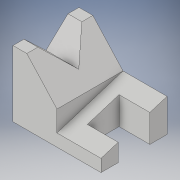
# Autodesk Inventor part: orthographic2
Saved by Autodesk Inventor 2017 (Build 210142000, 142)
## iProperties
Created: 2018-11-30
Part Number: orthographic2
Material: Generic
Document SubType Name: Modeling
Designer: qthuynh
Density: 1 g/cm^3
Appearance: Default
Author: qthuynh
Autodesk Inventor part; units mm, degrees
ref_plane "YZ Plane" through (0, 0, 0) normal (1, 0, 0) x (0, 1, 0)
ref_plane "XZ Plane" through (0, 0, 0) normal (0, 1, 0) x (-1, 0, 0)
ref_plane "XY Plane" through (0, 0, 0) normal (0, 0, 1) x (1, 0, 0)
sketch "Sketch1" plane through (0, 0, 0) normal (0, 0, 1) x (1, 0, 0)
  line L0 (0, 0) -> (101.6, 0)
  line L1 (101.6, 0) -> (101.6, 76.2)
  line L2 (101.6, 76.2) -> (0, 76.2)
  line L3 (0, 76.2) -> (0, 0)
  dimension "d0" = 101.6
  dimension "d1" = 76.2
  constraints: 8 end point, 2 parallel, 1 horizontal, 1 perpendicular
  measures "d0" distance of L2.end L1.end
  measures "d1" distance of L1.end L0.end
extrude "Extrusion1" add sketch "Sketch1" along normal blind 76.2
sketch "Sketch2" plane through (0, 76.2, 0) normal (0, 1, 0) x (1, 0, 0)
  line L0 (101.6, 0) -> (101.6, -76.2) projected
  line L1 (101.6, -19.812) -> (66.04, -19.812)
  line L2 (66.04, -19.812) -> (66.04, -56.388)
  line L3 (66.04, -56.388) -> (101.6, -56.388)
  line L4 (101.6, -56.388) -> (101.6, -19.812)
  point P0 (0, 0)
  dimension "d4" = 35.56
  dimension "d5" = 36.576
  dimension "d6" = 19.812
  constraints: 8 end point, 2 parallel, 1 horizontal, 1 perpendicular, 1 point on line
  measures "d4" distance of L3.end L2.end
  measures "d5" distance of L2.end L1.end
  measures "d6" distance of L0.start L1.start
extrude "Extrusion2" cut sketch "Sketch2" against normal blind 76.2
sketch "Sketch3" plane through (0, 0, 76.2) normal (0, 0, 1) x (1, 0, 0)
  line L0 (0, 75.8832) -> (15.9989, 76.2)
  line L1 (101.6, 76.2) -> (0, 76.2) projected
  line L2 (66.04, 0) -> (101.6, 0) projected
  line L3 (101.6, 0) -> (50.8, 0)
  line L4 (101.6, 0) -> (101.6, 38.1)
  line L5 (101.6, 76.2) -> (101.6, 0) projected
  line L6 (50.8, 0) -> (50.8, 38.1)
  line L7 (15.9989, 76.2) -> (50.8, 38.1)
  line L8 (101.6, 38.1) -> (101.6, 90.7152)
  line L9 (101.6, 90.7152) -> (15.9989, 90.7152)
  line L10 (15.9989, 90.7152) -> (15.9989, 76.2)
  line L11 (50.8, 38.1) -> (101.6, 38.1)
  point P0 (0, 0)
  dimension "d9" = 16.002
  dimension "d10" = 50.8
  dimension "d11" = 38.1
  constraints: 18 end point, 2 perpendicular, 2 point on line, 1 collinear, 1 horizontal, 1 midpoint, 1 vertical
  measures "d9" distance of L0.start L0.end
  measures "d10" distance of L2.end L3.end
  measures "d11" distance of L2.end L4.end
extrude "Extrusion3" cut sketch "Sketch3" against normal blind 76.2 contours L5 L11 L7 L1
sketch "Sketch4" plane through (101.6, 0, 76.2) normal (1, 0, 0) x (0, 0, -1)
  line L0 (76.2, 38.1) -> (56.388, 38.1) projected
  line L1 (0, 0) -> (0, 38.1) projected
  line L2 (76.2, 38.1) -> (0, 38.1)
  line L3 (0, 38.1) -> (0, 14.224)
  line L4 (0, 14.224) -> (76.2, 38.1)
  point P0 (76.2, 0)
  dimension "d14" = 23.876
  constraints: 6 end point, 1 horizontal, 1 point on line
  measures "d14" distance of L1.end L3.end
extrude "Extrusion4" cut sketch "Sketch4" against normal blind 50.8
sketch "Sketch5" plane through (0, 0, 0) normal (-1, 0, 0) x (0, 0, 1)
  point P0 (0, 0)
sketch "Sketch6" plane through (0, 0, 0) normal (-1, 0, 0) x (0, 0, 1)
  point P0 (0, 0)
sketch "Sketch7" plane through (0, 0, 0) normal (-1, 0, 0) x (0, 0, 1)
  line L0 (76.2, 76.2) -> (0, 76.2) projected
  line L1 (63.5, 76.2) -> (38.1, 76.2)
  line L2 (38.1, 76.2) -> (38.1, 52.324)
  line L3 (38.1, 52.324) -> (63.5, 76.2)
  line L4 (12.7, 76.2) -> (38.1, 76.2)
  line L5 (38.1, 52.324) -> (12.7, 76.2)
  line L6 (12.7, 76.2) -> (63.5, 76.2)
  point P0 (0, 0)
  dimension "d17" = 25.4
  dimension "d18" = 23.876
  dimension "d19" = 12.7
  constraints: 12 end point, 1 collinear, 1 midpoint, 1 perpendicular, 1 point on line, 1 symmetric about line
  measures "d17" distance of L1.start L1.end
  measures "d18" distance of L1.end L2.end
  measures "d19" distance of L0.end L5.end
sketch "Sketch8" plane through (0, 0, 0) normal (-1, 0, 0) x (0, 0, 1)
  point P0 (0, 0)
extrude "Extrusion5" cut sketch "Sketch7" against normal blind 50.8
body "Solid1"
